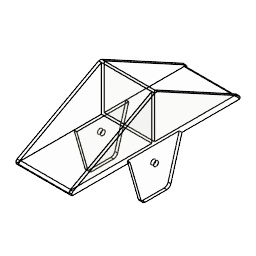
Bucket Receptacle (FA1) (Autodesk Fusion 360 design; units mm, degrees)
Autodesk Fusion 360 part; units mm, degrees
sketch "Sketch1" plane through (0, 0, 0) normal (0, 0, 1) x (1, 0, 0)
  line L0 (20, 60) -> (-20, 60)
  line L1 (-20, 60) -> (-20, -60)
  line L2 (-20, -60) -> (20, -60)
  line L3 (20, -60) -> (20, 60)
  line L4 (20, 60) -> (-20, -60) construction
  line L5 (-20, 60) -> (20, -60) construction
  dimension "d1" = 40
  dimension "d2" = 120
  constraint horizontal L0
  constraint perpendicular L0 L1
  constraint parallel L0 L2
  constraint parallel L1 L3
  constraint coincident L4 origin
  constraint coincident L5 origin
  measures "d1" distance of L1.end L2.end
  measures "d2" distance of L0.end L1.end
extrude "Extrude1" add sketch "Sketch1" along normal blind 2
sketch "Sketch2" plane through (0, 0, 0) normal (1, 0, 0) x (0, 1, 0)
  line L0 (-1, 2) -> (1, 2)
  line L1 (1, 2) -> (1, 34)
  line L2 (1, 34) -> (-1, 34)
  line L3 (-1, 34) -> (-1, 2)
  line L4 (-60, 2) -> (-1, 34)
  line L5 (-60, 2) -> (-1, 2)
  line L6 (1, 34) -> (60, 2)
  line L7 (1, 2) -> (60, 2)
  dimension "d5" = 32
  dimension "d16" = 2
  dimension "d25" = 1
  dimension "d26" = 60
  dimension "d27" = 2
  constraint horizontal L0
  constraint vertical L1
  constraint horizontal L2
  constraint vertical L3
  constraint perpendicular L3 L5
  constraint perpendicular L1 L7
  constraint equal L5 L7
  measures "d5" distance of L0.start L2.end
  measures "d16" distance of L0.start L0.end
  measures "d25" distance of origin L3
  measures "d26" horizontal distance of origin L6.end
  measures "d27" distance of origin L0
sketch "Sketch3" plane through (0, 0, 0) normal (1, 0, 0) x (0, 1, 0)
  line L0 (0, 0) -> (0, -30) construction
  line L1 (0, 0) -> (0, -10) construction
  circle A0 centre (0, -10) radius 1.75
  line L2 (0, -30) -> (-7.7353, -30)
  line L3 (-10.6205, -27.8219) -> (-18.5463, 0)
  line L4 (0, -30) -> (7.7353, -30)
  line L5 (10.6205, -27.8219) -> (18.5463, 0)
  line L6 (18.5463, 0) -> (-18.5463, 0)
  arc A1 (7.7353, -30) -> (10.6205, -27.8219) centre (7.7353, -27) ccw
  arc A2 (-10.6205, -27.8219) -> (-7.7353, -30) centre (-7.7353, -27) ccw
  dimension "d21" = 10
  dimension "d22" = 3.5
  dimension "d23" = 30
  dimension "d24" = 3
  dimension "d28" = 18.5463
  dimension "d29" = 74.099
  constraint coincident L0.start L1.start
  constraint vertical L0
  constraint coincident L1.end A0.centre
  constraint perpendicular L0 L2
  constraint symmetric L2.start L0 L4.start
  constraint symmetric L0 L3.end L5.end
  constraint tangent L4 A1
  constraint tangent L5 A1
  constraint tangent L2 A2
  constraint tangent L3 A2
  constraint equal A1 A2
  constraint vertical L0.start L1.end
  constraint symmetric L0 L5.start L3.start
  constraint coincident L0.start L6
  measures "d21" distance of L0.start L1.end
  measures "d22" diameter of A0
  measures "d23" distance of L0.start L0.end
  measures "d24" radius of A1
  measures "d28" distance of L0 L3.end
  measures "d29" angle of L5 L6
extrude "Extrude2" add sketch "Sketch2" along normal up to surface (20 mm away) and the other way up to surface (20 mm away) contours L0 L1 L2 L3
extrude "Extrude3" add sketch "Sketch2" sketch "Sketch3" against normal blind 2 of sketch 2 start surface through (20, -60, 0) normal (1, 0, 0)
extrude "Extrude4" add sketch "Sketch2" sketch "Sketch3" along normal blind 2 of sketch 2 start surface through (-20, 60, 0) normal (-1, 0, 0)
fillet "Fillet1" radius 1.5 6 edges at (0, 60, 2) (19, 60, 2) (-19, 60, 2) (0, -60, 2) (19, -60, 2) (-19, -60, 2)
